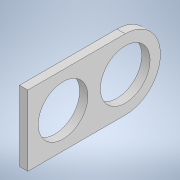
# Autodesk Inventor part: lamp_holder_front
Saved by Autodesk Inventor 2021 (Build 250183000, 183)
## iProperties
Created: 2020-12-10
Part Number: lamp_holder_front
Material: Generic
Document SubType Name: Modeling
Designer: Mateusz
Density: 1 g/cm^3
Appearance: Default
Author: Mateusz
Autodesk Inventor part; units mm, degrees
ref_plane "YZ Plane" through (0, 0, 0) normal (1, 0, 0) x (0, 1, 0)
ref_plane "XZ Plane" through (0, 0, 0) normal (0, 1, 0) x (-1, 0, 0)
ref_plane "XY Plane" through (0, 0, 0) normal (0, 0, 1) x (1, 0, 0)
sketch "Sketch1" plane through (0, 0, 0) normal (1, 0, 0) x (0, 1, 0)
  circle A0 centre (0, 0) radius 12
  circle A1 centre (0, -30) radius 12
  line L0 (17, -30) -> (17, 0)
  arc A2 (-17, -30) -> (17, -30) centre (0, -30) ccw
  line L1 (-17, -30) -> (-17, 12)
  line L2 (17, 12) -> (17, 0)
  line L3 (17, 12) -> (17, 17)
  line L4 (17, 17) -> (-17, 17)
  line L5 (-17, 17) -> (-17, 12)
  constraints: 12 end point, 3 centre point, 3 vertical, 2 point on circle, 1 coincident, 1 collinear, 1 perpendicular, 1 tangent
extrude "Extrusion1" add sketch "Sketch1" along normal blind 4
body "Solid1"
